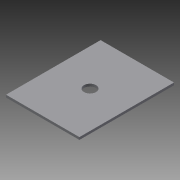
# Autodesk Inventor part: pcbProtectiveCaseTop
Saved by Autodesk Inventor 2015 (Build 190159000, 159)
## iProperties
Created: 2015-02-12
Part Number: pcbProtectiveCaseTop
Material: Generic
Document SubType Name: Modeling
Designer: 477grp12
Density: 1 g/cm^3
Appearance: Default
Mass: 9.38455 g
Surface Area: 100.044 cm^2
Volume: 9.38455 cm^3
Author: 477grp12
Autodesk Inventor part; units mm, degrees
ref_plane "YZ Plane" through (0, 0, 0) normal (1, 0, 0) x (0, 1, 0)
ref_plane "XZ Plane" through (0, 0, 0) normal (0, 1, 0) x (-1, 0, 0)
ref_plane "XY Plane" through (0, 0, 0) normal (0, 0, 1) x (1, 0, 0)
sketch "Sketch1" plane through (0, 0, 0) normal (0, 1, 0) x (-1, 0, 0)
  line L0 (60.86, 0) -> (0, 0)
  line L1 (0, 0) -> (0, -78.39)
  line L2 (0, -78.39) -> (60.86, -78.39)
  line L3 (60.86, -78.39) -> (60.86, 0)
  dimension "d0" = 78.39
  dimension "d1" = 60.86
  constraints: 8 end point, 2 parallel, 1 coincident, 1 horizontal, 1 perpendicular
  measures "d0" distance of L2.end L0.start
  measures "d1" distance of L1.end L2.end
extrude "Extrusion1" add sketch "Sketch1" along normal blind 2
sketch "Sketch2" plane through (0, 2, 0) normal (0, 1, 0) x (1, 0, 0)
  line L0 (0, 78.39) -> (-60.86, 78.39) projected
  line L1 (-60.86, 78.39) -> (-60.86, 0) projected
  point P0 (0, 0)
  point P1 (-30.43, 39.195)
  dimension "d4" = 39.195
  dimension "d5" = 30.43
  measures "d4" distance from line of L0 point (-30.43, 39.195)
  measures "d5" distance from line of L1 point (-30.43, 39.195)
hole "Hole1" at (-30.43, 2, -39.195) direction (0, -1, 0) diameter 10 end through all
body "Solid1"
